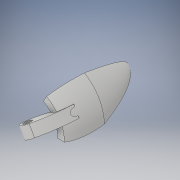
# Autodesk Inventor part: Innter_petal
Saved by Autodesk Inventor 2019 (Build 230136000, 136)
## iProperties
Created: 2019-11-16
Part Number: Innter_petal
Material: Generic
Document SubType Name: Modeling
Designer: Jorian Brusind
Density: 1 g/cm^3
Appearance: Default
Author: Jorian Brusind
Autodesk Inventor part; units mm, degrees
ref_plane "YZ Plane" through (0, 0, 0) normal (1, 0, 0) x (0, 1, 0)
sketch "Sketch1" plane through (0, 0, 0) normal (0, 1, 0) x (-1, 0, 0)
  line L0 (0, 0) -> (0, -30)
  line L1 (0, 0) -> (30, 0) construction
  spline S0 degree 2 poles (0, -30) (-5.2172, -27.9207) (-10.8719, -12.7372) knots 0 0 0 1 1 1
  line L2 (-10.8719, -12.7372) -> (-12.8062, 1.9407) construction
  line L3 (-12.8062, 1.9407) -> (0, 0) construction
  spline S1 degree 2 poles (-10.8719, -12.7372) (-12.8062, 1.9407) (0, 0) knots 1 1 1 2 2 2
  point P0 (-3.8105, -26.8078)
  dimension "d16" = 30
  dimension "d17" = 90
  constraints: 4 end point, 1 horizontal, 1 perpendicular, 1 vertical, 6 other
  measures "d16" distance of L0.start L0.end
  measures "d17" angle of L0 L1
revolve "Revolution3" add sketch "Sketch1" angle 60 about axis through (0, 0, 0) along (0, 0, 1)
sketch "Sketch6" plane through (0, 0, -30) normal (0, -1, 0) x (1, 0, 0)
  line L0 (0, 30) -> (0, 27)
  line L1 (0, 30) -> (0, 0) projected
  line L2 (0, 27) -> (15, 27)
  line L3 (0, 0) -> (0, 1.5)
  spline S0 degree 3 poles (0, 1.5) (5.1775, 3.9151) (12.4804, 18.8279) (7.9089, 27) knots 0 0 0 0 1 1 1 1
  point P0 (4.4382, 5.8918)
  point P1 (8.9326, 16.7012)
  dimension "d19" = 3
  dimension "d20" = 15
  dimension "d21" = 1.5
  constraints: 6 end point, 3 point on line, 1 perpendicular, 4 other
  measures "d19" distance of L0.start L0.end
  measures "d20" distance of L0.end L2.end
  measures "d21" distance of L1.end L3.end
revolve "Revolution4" cut sketch "Sketch6" angle 360 about axis through (0, 0, 0) along (0, 0, -1)
sketch "Sketch7" plane through (0, 0, -3) normal (0, -1, 0) x (1, 0, 0)
  line L0 (0, 3) -> (0, 0) projected
  line L1 (0, 0) -> (13, 0)
  line L2 (13, 0) -> (13, 5)
  line L3 (13, 5) -> (0, 5)
  line L4 (0, 5) -> (0, 0)
  dimension "d23" = 13
  dimension "d24" = 5
  constraints: 8 end point, 2 parallel, 1 horizontal, 1 perpendicular
  measures "d23" distance of L3.end L2.end
  measures "d24" distance of L2.end L1.end
revolve "Revolution5" cut sketch "Sketch7" angle 360 about axis through (0, 0, 0) along (0, 0, -1)
sketch "Sketch8" plane through (0, 0, -30) normal (-0.866, 0.5, 0) x (0, 0, 1)
  line L0 (1.5, 0) -> (0, 0) projected
  line L1 (1.5, 0) -> (30, 0)
  constraints: 2 end point, 1 horizontal
ref_plane "Work Plane2" through (0, 0, -28.5) normal (0.5, -0.866, 0) x (0, 0, 1)
sketch "Sketch9" plane through (0, 0, -28.5) normal (0.5, -0.866, 0) x (0, 0, 1)
  line L0 (25.5, -6.8493) -> (25.5, -8.3976) projected
  line L1 (25.5, -7.9089) -> (25.5, -6.8493) projected
  line L2 (25.5, -8.3976) -> (25.5, -7.9089)
  line L3 (25.5, -7.9089) -> (25.5, -13.2779)
  line L4 (25.5, -7.9089) -> (29.8301, -5.4089)
  line L5 (25.5, -7.9089) -> (30.5, -7.9089) construction
  circle A0 centre (29.8301, -5.4089) radius 1.75
  circle A1 centre (29.8301, -5.4089) radius 1.05
  spline S0 degree 2 poles (30.7051, -6.9244) (27.615, -9.9944) (21.9704, -10.8927) knots 0 0 0 1 1 1
  spline S1 degree 3 poles (28.9551, -3.8934) (23.9976, -6.7492) (23.8027, -11.1988) (20.2008, -10.2065) knots 0 0 0 0 1 1 1 1
  line L6 (21.9704, -10.8927) -> (20.2008, -10.2065)
  point P0 (28.5, 0)
  point P1 (27.284, -9.3075)
  point P2 (24.5466, -7.9089)
  point P3 (22.5368, -9.9569)
  dimension "d27" = 5
  dimension "d28" = 30
  dimension "d29" = 3.5
  dimension "d30" = 2.1
  constraints: 10 end point, 2 centre point, 2 coincident, 2 point on circle, 1 equal length, 1 horizontal, 1 point on line, 1 vertical, 7 other
  measures "d27" distance of L1.start L4.end
  measures "d28" angle of L5 L4
  measures "d29" diameter of A0
  measures "d30" diameter of A1
extrude "Extrusion2" add sketch "Sketch9" along normal mid plane 3
ref_plane "Work Plane3" through (0, 0, -28.5) normal (1, 0, 0) x (0, 0, 1)
body "Solid2"
